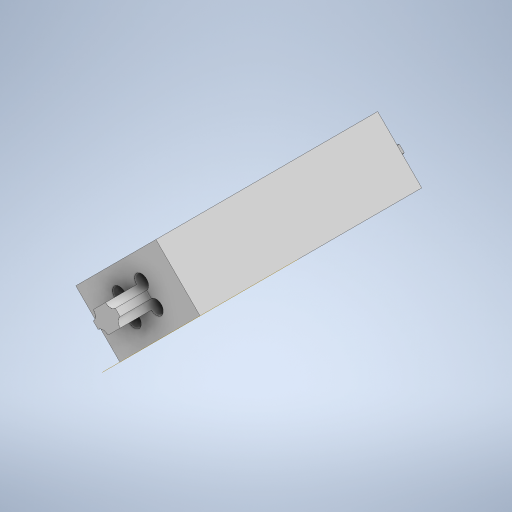
# Autodesk Inventor part: _armpit_adt_2
Saved by Autodesk Inventor 2024.3 (Build 283343000, 343)
## iProperties
Created: 2024-09-06
Part Number: _armpit_adt_2
Material: 일반
Document SubType Name: Modeling
Designer: gretc
Density: 1 g/cm^3
Appearance: 기본값
Author: gretc
Autodesk Inventor part; units mm, degrees
ref_plane "YZ Plane" through (0, 0, 0) normal (1, 0, 0) x (0, 1, 0)
ref_plane "XZ Plane" through (0, 0, 0) normal (0, 1, 0) x (-1, 0, 0)
ref_plane "XY Plane" through (0, 0, 0) normal (0, 0, 1) x (1, 0, 0)
ref_plane "작업 평면1" through (0, 0, -6) normal (0, 0, -1) x (-1, 0, 0)
sketch "스케치1" plane through (0, 0, -6) normal (0, 0, -1) x (-1, 0, 0)
  arc A0 (7.7127, 5.3793) -> (9.6219, 5.3793) centre (8.6673, 4.4247) ccw projected
  line L0 (7.7127, 5.3793) -> (5.3793, 7.7127) projected
  arc A1 (5.3793, 9.6219) -> (5.3793, 7.7127) centre (4.4247, 8.6673) ccw projected
  line L1 (5.3793, 9.6219) -> (6.2985, 10.5412) projected
  arc A2 (8.2077, 10.5412) -> (6.2985, 10.5412) centre (7.2531, 11.4958) ccw projected
  line L2 (8.2077, 10.5412) -> (10.5412, 8.2077) projected
  arc A3 (10.5412, 6.2985) -> (10.5412, 8.2077) centre (11.4958, 7.2531) ccw projected
  line L3 (10.5412, 6.2985) -> (9.6219, 5.3793) projected
  line L4 (-11.8741, -6.1466) -> (-19.0298, -13.3022) projected
  arc A4 (-6.1466, -11.8741) -> (-11.8741, -6.1466) centre (-9.0103, -9.0103) ccw projected
  line L5 (-13.3022, -19.0298) -> (-6.1466, -11.8741) projected
  arc A5 (-13.3022, -19.0298) -> (-1.3029, -16.7178) centre (-9.0103, -9.0103) ccw projected
  line L6 (19.9103, 4.4954) -> (-1.3029, -16.7178) projected
  line L7 (4.4954, 19.9103) -> (19.9103, 4.4954) projected
  line L8 (-16.7178, -1.3029) -> (4.4954, 19.9103) projected
  arc A6 (-16.7178, -1.3029) -> (-19.0298, -13.3022) centre (-9.0103, -9.0103) ccw projected
  circle A7 centre (-9.0103, -17.0103) radius 1.2 projected
  circle A8 centre (-14.6672, -3.3535) radius 1.2 projected
  circle A9 centre (-17.0103, -9.0103) radius 1.2 projected
  circle A10 centre (-1.0103, -9.0103) radius 1.2 projected
  circle A11 centre (-9.0103, -1.0103) radius 1.2 projected
  circle A12 centre (-3.3535, -3.3535) radius 1.2 projected
  circle A13 centre (-3.3535, -14.6672) radius 1.2 projected
  line L9 (4.4247, 8.6673) -> (-1.1614, 14.2535)
  line L10 (7.2531, 11.4958) -> (1.667, 17.0819)
  line L11 (8.6673, 4.4247) -> (14.2535, -1.1614)
  circle A14 centre (4.4247, 8.6673) radius 1.35
  circle A15 centre (8.6673, 4.4247) radius 1.35
  circle A16 centre (11.4958, 7.2531) radius 1.35
  circle A17 centre (7.2531, 11.4958) radius 1.35
  point P0 (0, 0)
  point P1 (5.3793, 9.6219)
  point P2 (9.6219, 5.3793)
  point P3 (10.5412, 6.2985)
  constraints: 6 end point, 4 coincident, 4 point on line, 2 perpendicular, 12 other
extrude "돌출1" add sketch "스케치1" against normal blind 54.65 contours A15 L0 A14 L1 A17 L2 A16 L3
ref_plane "작업 평면2" through (0, 0, 0) normal (0, 0, 1) x (1, 0, 0)
sketch "스케치2" plane through (0, 0, 0) normal (0, 0, 1) x (1, 0, 0)
  arc A0 (-9.6219, 5.3793) -> (-7.7127, 5.3793) centre (-8.6673, 4.4247) ccw projected
  line L0 (-9.6219, 5.3793) -> (-10.5412, 6.2985) projected
  arc A1 (-10.5412, 8.2077) -> (-10.5412, 6.2985) centre (-11.4958, 7.2531) ccw projected
  line L1 (-10.5412, 8.2077) -> (-8.2077, 10.5412) projected
  arc A2 (-6.2985, 10.5412) -> (-8.2077, 10.5412) centre (-7.2531, 11.4958) ccw projected
  line L2 (-6.2985, 10.5412) -> (-5.3793, 9.6219) projected
  arc A3 (-5.3793, 7.7127) -> (-5.3793, 9.6219) centre (-4.4247, 8.6673) ccw projected
  line L3 (-5.3793, 7.7127) -> (-7.7127, 5.3793) projected
  line L4 (11.8741, -6.1466) -> (19.0298, -13.3022) projected
  arc A4 (19.0298, -13.3022) -> (16.7178, -1.3029) centre (9.0103, -9.0103) ccw projected
  line L5 (16.7178, -1.3029) -> (-4.4954, 19.9103) projected
  line L6 (-4.4954, 19.9103) -> (-19.9103, 4.4954) projected
  line L7 (-19.9103, 4.4954) -> (1.3029, -16.7178) projected
  arc A5 (1.3029, -16.7178) -> (13.3022, -19.0298) centre (9.0103, -9.0103) ccw projected
  line L8 (13.3022, -19.0298) -> (6.1466, -11.8741) projected
  arc A6 (11.8741, -6.1466) -> (6.1466, -11.8741) centre (9.0103, -9.0103) ccw projected
  circle A7 centre (9.0103, -17.0103) radius 1.2 projected
  circle A8 centre (14.6672, -3.3535) radius 1.2 projected
  circle A9 centre (17.0103, -9.0103) radius 1.2 projected
  circle A10 centre (1.0103, -9.0103) radius 1.2 projected
  circle A11 centre (9.0103, -1.0103) radius 1.2 projected
  circle A12 centre (3.3535, -3.3535) radius 1.2 projected
  circle A13 centre (3.3535, -14.6672) radius 1.2 projected
  line L9 (-5.3793, 9.6219) -> (-6.2985, 10.5412) projected
  arc A14 (-8.2077, 10.5412) -> (-6.2985, 10.5412) centre (-7.2531, 11.4958) ccw projected
  line L10 (-8.2077, 10.5412) -> (-10.5412, 8.2077) projected
  arc A15 (-10.5412, 6.2985) -> (-10.5412, 8.2077) centre (-11.4958, 7.2531) ccw projected
  line L11 (-10.5412, 6.2985) -> (-9.6219, 5.3793) projected
  arc A16 (-7.7127, 5.3793) -> (-9.6219, 5.3793) centre (-8.6673, 4.4247) ccw projected
  line L12 (-7.7127, 5.3793) -> (-5.3793, 7.7127) projected
  arc A17 (-5.3793, 9.6219) -> (-5.3793, 7.7127) centre (-4.4247, 8.6673) ccw projected
  line L13 (-4.4954, 19.9103) -> (-19.9103, 4.4954)
  line L14 (-19.9103, 4.4954) -> (-11.4251, -3.9899)
  line L15 (-11.4251, -3.9899) -> (3.9899, 11.4251)
  line L16 (3.9899, 11.4251) -> (-4.4954, 19.9103)
  point P0 (0, 0)
  point P1 (3.9899, 11.4251)
  dimension "d2" = 12
  constraints: 8 end point, 2 parallel, 2 perpendicular
  measures "d2" distance of L14.end L6.end
ref_plane "작업 평면3" through (3.9899, 11.4251, 42.65) normal (0.7071068, -0.7071068, 0) x (-0.7071068, -0.7071068, 0)
extrude "돌출3" add sketch "스케치2" along normal blind 42.65 contours L15 L7 L6 L5
sketch "스케치5" plane through (-19.9103, 4.4954, 0) normal (-0.7071068, 0.7071068, 0) x (-0.7071068, -0.7071068, 0)
  line L0 (-15.25, 42.65) -> (-15.25, 0) projected
  line L1 (-12.55, 48.65) -> (-12.55, -6) projected
  line L2 (-9.25, 48.65) -> (-9.25, -6) projected
  line L3 (-6.55, 42.65) -> (-6.55, 0) projected
  line L4 (-6.55, 0) -> (-6.55, 4)
  line L5 (-6.55, 4) -> (-9.25, 4)
  line L6 (-15.25, 0) -> (-15.25, 4)
  line L7 (-15.25, 4) -> (-12.55, 4)
  line L8 (-9.9, 5) -> (-5.9, 5)
  line L9 (-5.9, 5) -> (-5.9, 3)
  line L10 (-5.9, 3) -> (-9.9, 3)
  line L11 (-9.9, 3) -> (-9.9, 5)
  line L12 (-9.9, 5) -> (-5.9, 3) construction
  line L13 (-5.9, 5) -> (-9.9, 3) construction
  line L14 (-15.9579, 5) -> (-11.8421, 5)
  line L15 (-11.8421, 5) -> (-11.8421, 3)
  line L16 (-11.8421, 3) -> (-15.9579, 3)
  line L17 (-15.9579, 3) -> (-15.9579, 5)
  line L18 (-15.9579, 5) -> (-11.8421, 3) construction
  line L19 (-11.8421, 5) -> (-15.9579, 3) construction
  line L20 (-6.55, 42.65) -> (-6.55, 38.65)
  line L21 (-6.55, 38.65) -> (-15.25, 38.65)
  line L22 (-9.25, 38.65) -> (-7.9, 38.65)
  line L23 (-12.55, 38.65) -> (-13.9, 38.65)
  line L24 (-9.9, 39.65) -> (-5.9, 39.65)
  line L25 (-5.9, 39.65) -> (-5.9, 37.65)
  line L26 (-5.9, 37.65) -> (-9.9, 37.65)
  line L27 (-9.9, 37.65) -> (-9.9, 39.65)
  line L28 (-9.9, 39.65) -> (-5.9, 37.65) construction
  line L29 (-5.9, 39.65) -> (-9.9, 37.65) construction
  line L30 (-15.9, 39.65) -> (-11.9, 39.65)
  line L31 (-11.9, 39.65) -> (-11.9, 37.65)
  line L32 (-11.9, 37.65) -> (-15.9, 37.65)
  line L33 (-15.9, 37.65) -> (-15.9, 39.65)
  line L34 (-15.9, 39.65) -> (-11.9, 37.65) construction
  line L35 (-11.9, 39.65) -> (-15.9, 37.65) construction
  point P0 (-10.9, 0)
  point P1 (-7.9, 4)
  point P2 (-13.9, 4)
  dimension "d7" = 4
  dimension "d8" = 4
  dimension "d9" = 2
  dimension "d10" = 2
  dimension "d13" = 4
  dimension "d14" = 4
  dimension "d15" = 2
  dimension "d16" = 4
  constraints: 64 end point, 12 point on line, 10 midpoint, 8 parallel, 7 perpendicular, 2 coincident, 1 horizontal
  measures "d7" distance of L3.end L4.end
  measures "d8" distance of L8.start L8.end
  measures "d9" distance of L8.end L9.end
  measures "d10" distance of L14.end L15.end
  measures "d13" distance of L3.start L20.end
  measures "d14" distance of L24.start L24.end
  measures "d15" distance of L24.end L25.end
  measures "d16" distance of L30.start L30.end
extrude "돌출4" cut sketch "스케치5" against normal blind 4 contours L30 L1 L21 L0 | L0 L32 L33 L30 | L21 L1 L32 L0 | L30 L31 L21 L1 | L21 L31 L32 L1 | L14 L1 L7 L0 | L0 L16 L17 L14 | L7 L1 L16 L0 | L14 L15 L16 L1 | L24 L3 L21 L2 | L2 L21 L27 L24 | L21 L3 L26 L2 | L2 L26 L27 L21 | L24 L25 L26 L3 | L8 L3 L5 L2 | L2 L10 L11 L8 | L5 L3 L10 L2 | L8 L9 L10 L3
